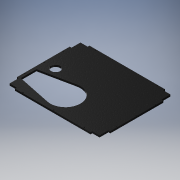
# Autodesk Inventor part: top
Saved by Autodesk Inventor 2018 (Build 220112000, 112)
## iProperties
Created: 2017-10-09
Part Number: top
Material: Generic
Document SubType Name: Modeling
Designer: HP
Density: 1 g/cm^3
Appearance: Fine Textured - Black
Author: HP
Autodesk Inventor part; units mm, degrees
ref_plane "YZ Plane" through (0, 0, 0) normal (1, 0, 0) x (0, 1, 0)
ref_plane "XZ Plane" through (0, 0, 0) normal (0, 1, 0) x (-1, 0, 0)
ref_plane "XY Plane" through (0, 0, 0) normal (0, 0, 1) x (1, 0, 0)
sketch "Sketch1" plane through (0, 0, 0) normal (0, 0, 1) x (1, 0, 0)
  line L0 (-236.1, 0) -> (-211.1, 0) construction
  line L1 (-211.1, 0) -> (-211.1, 5) construction
  line L2 (-236.1, 5) -> (-211.1, 5) construction
  line L3 (-236.1, 0) -> (-236.1, 5) construction
  circle A0 centre (-21.1, 2.5) radius 1.2295 construction
  circle A1 centre (-106.1, 2.5) radius 1.2295 construction
  circle A2 centre (-191.1, 2.5) radius 1.2295 construction
  line L4 (-211.1, 0) -> (0, 0) construction
  line L5 (-1.1, 0) -> (-1.1, 5) construction
  line L6 (-211.1, 5) -> (-1.1, 5) construction
  line L7 (-211.1, 0) -> (-211.1, 5) construction
  line L8 (0, 0) -> (23.9, 0) construction
  line L9 (23.9, 0) -> (23.9, 5) construction
  line L10 (-1.1, 5) -> (23.9, 5) construction
  line L11 (-1.1, 0) -> (-1.1, 5) construction
  line L12 (18.9, 0) -> (18.9, -25) construction
  line L13 (18.9, -25) -> (23.9, -25) construction
  line L14 (23.9, 0) -> (23.9, -25) construction
  line L15 (18.9, 0) -> (23.9, 0) construction
  circle A3 centre (21.4, -45) radius 1.2295 construction
  circle A4 centre (21.4, -98.5) radius 1.2295 construction
  circle A5 centre (21.4, -152) radius 1.2295 construction
  line L16 (18.9, -25) -> (18.9, -172) construction
  line L17 (18.9, -172) -> (23.9, -172) construction
  line L18 (23.9, -25) -> (23.9, -172) construction
  line L19 (18.9, -25) -> (23.9, -25) construction
  line L20 (-236.1, 0) -> (-236.1, -25) construction
  line L21 (-236.1, -25) -> (-231.1, -25) construction
  line L22 (-231.1, 0) -> (-231.1, -25) construction
  line L23 (-236.1, 0) -> (-231.1, 0) construction
  circle A6 centre (-233.6, -45) radius 1.2295 construction
  circle A7 centre (-233.6, -98.5) radius 1.2295 construction
  circle A8 centre (-233.6, -152) radius 1.2295 construction
  line L24 (-236.1, -25) -> (-236.1, -172) construction
  line L25 (-236.1, -172) -> (-231.1, -172) construction
  line L26 (-231.1, -25) -> (-231.1, -172) construction
  line L27 (-236.1, -25) -> (-231.1, -25) construction
  line L28 (-236.1, -172) -> (-236.1, -197) construction
  line L29 (-236.1, -197) -> (-231.1, -197) construction
  line L30 (-231.1, -172) -> (-231.1, -197) construction
  line L31 (-236.1, -172) -> (-231.1, -172) construction
  line L32 (-211.1, -197) -> (-236.1, -197) construction
  line L33 (-236.1, -197) -> (-236.1, -202) construction
  line L34 (-211.1, -202) -> (-236.1, -202) construction
  line L35 (-211.1, -197) -> (-211.1, -202) construction
  circle A9 centre (-191.1, -199.5) radius 1.2295 construction
  circle A10 centre (-106.1, -199.5) radius 1.2295 construction
  circle A11 centre (-21.1, -199.5) radius 1.2295 construction
  line L36 (-1.1, -197) -> (-211.1, -197) construction
  line L37 (-211.1, -197) -> (-211.1, -202) construction
  line L38 (-1.1, -202) -> (-211.1, -202) construction
  line L39 (-1.1, -197) -> (-1.1, -202) construction
  line L40 (23.9, -197) -> (-1.1, -197) construction
  line L41 (-1.1, -197) -> (-1.1, -202) construction
  line L42 (23.9, -202) -> (-1.1, -202) construction
  line L43 (23.9, -197) -> (23.9, -202) construction
  line L44 (18.9, -172) -> (18.9, -197) construction
  line L45 (18.9, -197) -> (23.9, -197) construction
  line L46 (23.9, -172) -> (23.9, -197) construction
  line L47 (18.9, -172) -> (23.9, -172) construction
  line L48 (-1.1, -202) -> (-211.1, -202)
  line L49 (-211.1, -197) -> (-231.1, -197)
  line L50 (-231.1, -197) -> (-231.1, -172)
  line L51 (-236.1, -172) -> (-236.1, -25)
  line L52 (-231.1, -25) -> (-231.1, 0)
  line L53 (-231.1, 0) -> (-211.1, 0)
  line L54 (-211.1, 5) -> (-1.1, 5)
  line L55 (0, 0) -> (18.9, 0)
  line L56 (18.9, 0) -> (18.9, -25)
  line L57 (23.9, -25) -> (23.9, -172)
  line L58 (18.9, -172) -> (18.9, -197)
  line L59 (18.9, -197) -> (-1.1, -197)
  line L60 (-236.1, -172) -> (-231.1, -172)
  line L61 (-211.1, -197) -> (-211.1, -202)
  line L62 (-1.1, -202) -> (-1.1, -197)
  line L63 (18.9, -172) -> (23.9, -172)
  line L64 (18.9, -172) -> (18.9, -172)
  line L65 (18.9, -25) -> (23.9, -25)
  line L66 (18.9, -25) -> (18.9, -25)
  line L67 (-1.1, 5) -> (-1.1, 0)
  line L68 (-1.1, 0) -> (0, 0)
  line L69 (-211.1, 5) -> (-211.1, 0)
  line L70 (-211.1, 0) -> (-211.1, 0)
  line L71 (-236.1, -25) -> (-231.1, -25)
  line L72 (-231.1, -25) -> (-231.1, -25)
  dimension "d0" = 0
  dimension "d1" = 0
  dimension "d2" = 0
  dimension "d3" = 0
  dimension "d4" = 0
  dimension "d5" = 0
  dimension "d6" = 0
  dimension "d7" = 0
  constraints: 50 end point, 14 collinear, 14 point on line, 9 perpendicular, 1 horizontal
  measures "d0" distance between parallel lines of L25 L60
  measures "d1" distance between parallel lines of L35 L61
  measures "d2" distance between parallel lines of L41 L62
  measures "d3" distance between parallel lines of L17 L63
  measures "d4" distance between parallel lines of L13 L65
  measures "d5" distance between parallel lines of L5 L67
  measures "d6" distance between parallel lines of L1 L69
  measures "d7" distance between parallel lines of L21 L71
extrude "Extrusion1" add sketch "Sketch1" against normal blind 5
sketch "Sketch2" plane through (0, 0, 0) normal (0, 0, 1) x (1, 0, 0)
  circle A0 centre (-21.1, -199.5) radius 1.2295 construction
  circle A1 centre (-106.1, -199.5) radius 1.2295 construction
  circle A2 centre (-191.1, -199.5) radius 1.2295 construction
  circle A3 centre (-233.6, -152) radius 1.2295 construction
  circle A4 centre (-233.6, -98.5) radius 1.2295 construction
  circle A5 centre (-233.6, -45) radius 1.2295 construction
  circle A6 centre (-191.1, 2.5) radius 1.2295 construction
  circle A7 centre (-106.1, 2.5) radius 1.2295 construction
  circle A8 centre (-21.1, 2.5) radius 1.2295 construction
  circle A9 centre (21.4, -45) radius 1.2295 construction
  circle A10 centre (21.4, -98.5) radius 1.2295 construction
  circle A11 centre (21.4, -152) radius 1.2295 construction
  point P0 (0, 0)
hole "Hole1" at (-233.6, -152, 0) at (-233.6, -98.5, 0) at (-233.6, -45, 0) at (-191.1, 2.5, 0) at (-191.1, -199.5, 0) at (-106.1, -199.5, 0) at (-21.1, -199.5, 0) at (21.4, -152, 0) at (21.4, -98.5, 0) at (21.4, -45, 0) at (-106.1, 2.5, 0) at (-21.1, 2.5, 0) direction (0, 0, -1) diameter 3 end through all
sketch "Sketch3" plane through (0, 0, 0) normal (0, 0, 1) x (1, 0, 0)
  line L0 (-226.1, -127) -> (-226.1, -167) construction
  line L1 (-226.1, -167) -> (-134.2686, -186.157) construction
  arc A0 (-134.2686, -186.157) -> (-134.2686, -107.843) centre (-126.1, -147) ccw construction
  line L2 (-134.2686, -107.843) -> (-226.1, -127) construction
  line L3 (-134.677, -188.1149) -> (-228.1, -168.6258)
  line L4 (-228.1, -168.6258) -> (-228.1, -125.3742)
  line L5 (-228.1, -125.3742) -> (-134.677, -105.8851)
  arc A1 (-134.677, -188.1149) -> (-134.677, -105.8851) centre (-126.1, -147) ccw
  circle A2 centre (-203.1, -97) radius 12.5
  point P0 (0, 0)
  dimension "d17" = 2
  dimension "d18" = 50
  dimension "d19" = 25
  dimension "d20" = 25
  constraints: 6 end point, 2 centre point, 2 point on circle, 3 other
  measures "d17" distance between parallel lines of L1 L3
  measures "d18" vertical distance of A0.centre A2.centre
  measures "d19" distance from line of A2.centre L4
  measures "d20" diameter of A2
extrude "Extrusion2" [suppressed]
equation "\"d8\" = plate_thickness"
equation "\"plate_thickness\" = 5"
equation "\"basic_plate_offset\" = 0"
equation "\"ABS_tolerance\" = 0"
equation "\"laser_cutter_thickness\" = 0.1"
body "Solid1"
